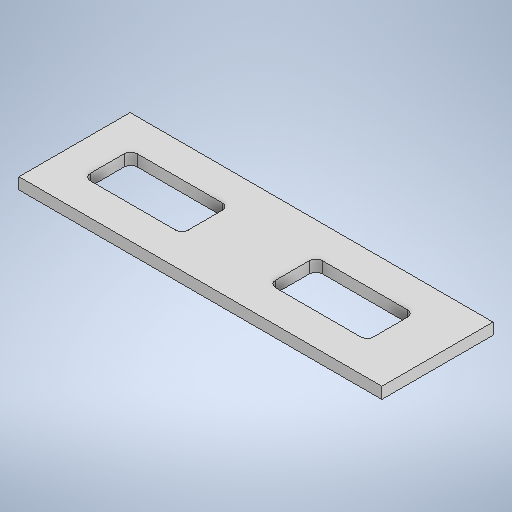
# Autodesk Inventor part: arcade_lid_extrusion_3.5
Saved by Autodesk Inventor 2025.2 (Build 292293000, 293)
## iProperties
Created: 2025-04-01
Part Number: arcade_lid_extrusion_3.5
Material: Generic
Document SubType Name: Modeling
Designer: osmon
Density: 1 g/cm^3
Appearance: Default
Author: osmon
Autodesk Inventor part; units mm, degrees
ref_plane "YZ Plane" through (0, 0, 0) normal (1, 0, 0) x (0, 1, 0)
ref_plane "XZ Plane" through (0, 0, 0) normal (0, 1, 0) x (-1, 0, 0)
ref_plane "XY Plane" through (0, 0, 0) normal (0, 0, 1) x (1, 0, 0)
sketch "Sketch1" plane through (0, 0, 0) normal (0, 1, 0) x (-1, 0, 0)
  line L0 (0, 0) -> (-111, 0)
  line L1 (-111, 0) -> (-111, -34)
  line L2 (-111, -34) -> (0, -34)
  line L3 (0, -34) -> (0, 0)
  dimension "d0" = 111
  dimension "d1" = 34
  constraints: 8 end point, 2 parallel, 1 horizontal, 1 perpendicular
  measures "d0" distance of L2.end L1.end
  measures "d1" distance of L1.end L0.end
extrude "Extrusion1" add sketch "Sketch1" along normal blind 3.5
sketch "Sketch2" plane through (0, 3.5, 0) normal (0, 1, 0) x (1, 0, 0)
  line L0 (10, 9.825) -> (40, 9.825)
  line L1 (40, 9.825) -> (40, 24.175)
  line L2 (40, 24.175) -> (10, 24.175)
  line L3 (10, 24.175) -> (10, 9.825)
  line L4 (66.65, 9.825) -> (96.65, 9.825)
  line L5 (96.65, 9.825) -> (96.65, 24.175)
  line L6 (96.65, 24.175) -> (66.65, 24.175)
  line L7 (66.65, 24.175) -> (66.65, 9.825)
  point P0 (0, 0)
  point P1 (66.65, 17)
  dimension "d4" = 30
  dimension "d5" = 14.35
  dimension "d6" = 30
  dimension "d7" = 14.35
  dimension "d8" = 26.65
  constraints: 16 end point, 4 parallel, 2 horizontal, 2 perpendicular, 1 midpoint, 1 point on line
  measures "d4" distance of L2.end L1.end
  measures "d5" distance of L1.end L0.end
  measures "d6" distance of L6.end L5.end
  measures "d7" distance of L5.end L4.end
  measures "d8" distance from line of point (66.65, 17) L1
extrude "Extrusion2" cut sketch "Sketch2" against normal blind 3.5
fillet "Fillet1" radius 2 8 edges at (10, 1.75, -24.175) (40, 1.75, -24.175) (10, 1.75, -9.825) (40, 1.75, -9.825) (66.65, 1.75, -9.825) (66.65, 1.75, -24.175) (96.65, 1.75, -9.825) (96.65, 1.75, -24.175)
body "Solid1"
